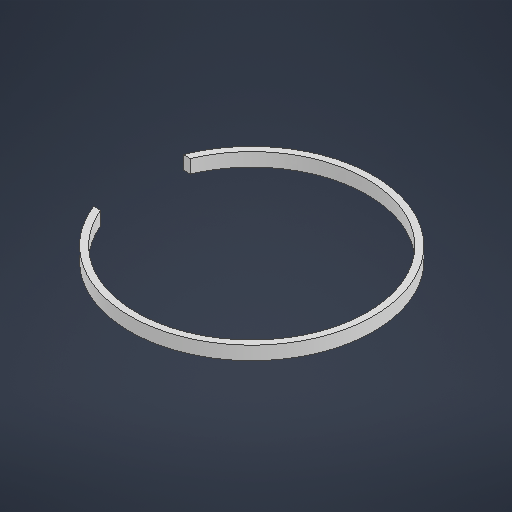
# Autodesk Inventor part: LEDs
Saved by Autodesk Inventor 2026.1 (Build 301233020, 233B)
## iProperties
Created: 2026-01-22
Part Number: LEDs
Material: Generic
Document SubType Name: Modeling
Designer: jacob
Density: 1 g/cm^3
Appearance: Default
Author: jacob
Autodesk Inventor part; units mm, degrees
ref_plane "YZ Plane" through (0, 0, 0) normal (1, 0, 0) x (0, 1, 0)
ref_plane "XZ Plane" through (0, 0, 0) normal (0, 1, 0) x (-1, 0, 0)
ref_plane "XY Plane" through (0, 0, 0) normal (0, 0, 1) x (1, 0, 0)
sketch "Sketch1" plane through (0, 0, 0) normal (0, 1, 0) x (-1, 0, 0)
  arc A0 (82.9156, 35) -> (82.9156, -35) centre (0, 0) ccw
  arc A1 (88.3176, 35) -> (88.3176, -35) centre (0, 0) ccw
  line L0 (0, 0) -> (0, -35)
  line L1 (0, 0) -> (0, 35)
  line L2 (82.9156, 35) -> (88.3176, 35)
  line L3 (82.9156, -35) -> (88.3176, -35)
  dimension "d1" = 180
  dimension "d2" = 190
  dimension "d3" = 35
  dimension "d4" = 35
  constraints: 8 end point, 4 point on circle, 2 centre point, 2 coincident, 2 vertical, 1 horizontal, 1 perpendicular
  measures "d1" diameter of A0
  measures "d2" diameter of A1
  measures "d3" distance of L0.start L0.end
  measures "d4" distance of L0.start L1.end
extrude "Extrusion1" add sketch "Sketch1" along normal blind 10.5
body "Solid1"
